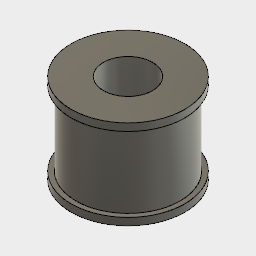
Idler Wheel (Autodesk Fusion 360 design; units mm, degrees)
Autodesk Fusion 360 part; units mm, degrees
sketch "Hub" plane through (0, 0, 0) normal (0, 1, 0) x (1, 0, 0)
  circle A0 centre (0, 0) radius 8.89
  dimension "d8" = 17.78
  measures "d8" diameter of A0
extrude "Extrude1" add sketch "Hub" along normal blind 15.24
sketch "Inner Cap" plane through (0, 0, 0) normal (0, -1, 0) x (1, 0, 0)
  circle A0 centre (0, 0) radius 8.89
  circle A1 centre (0, 0) radius 9.7155
  dimension "d11" = 19.431
  measures "d11" diameter of A1
extrude "Extrude2" add sketch "Inner Cap" against normal blind 1.27 contours A0 | A1
sketch "Outer Cap" plane through (0, 15.24, 0) normal (0, 1, 0) x (-1, 0, 0)
  circle A0 centre (0, 0) radius 8.89
  circle A1 centre (0, 0) radius 9.7155
  circle A2 centre (0, 0) radius 9.7155
  circle A3 centre (0, 0) radius 9.7155
extrude "Extrude3" add sketch "Outer Cap" against normal blind 1.27 contours A0 | A1 A2 A3
sketch "Bore" plane through (0, 15.24, 0) normal (0, 1, 0) x (-1, 0, 0)
  circle A0 centre (0, 0) radius 9.7155
  circle A1 centre (0, 0) radius 4.191
  dimension "d16" = 8.382
  measures "d16" diameter of A1
extrude "Extrude4" cut sketch "Bore" against normal blind 12.065 contours A1
sketch "Screw Hole" plane through (0, 15.24, 0) normal (0, 1, 0) x (-1, 0, 0)
  circle A0 centre (0, 0) radius 1.524
  dimension "d19" = 3.048
  measures "d19" diameter of A0
extrude "Extrude5" cut sketch "Screw Hole" against normal blind 72.644
equation "hubDia = 0.7 in"
equation "boreDia = 0.33 in"
equation "boreDepth = 0.475 in"
equation "screwHole = 0.12 in"
equation "capEndDia = 0.765 in"
equation "capThickness = 0.05 in"
equation "d8 = hubDia"
equation "d11 = capEndDia"
equation "d16 = boreDia"
equation "d17 = -boreDepth"
equation "d19 = screwHole"
